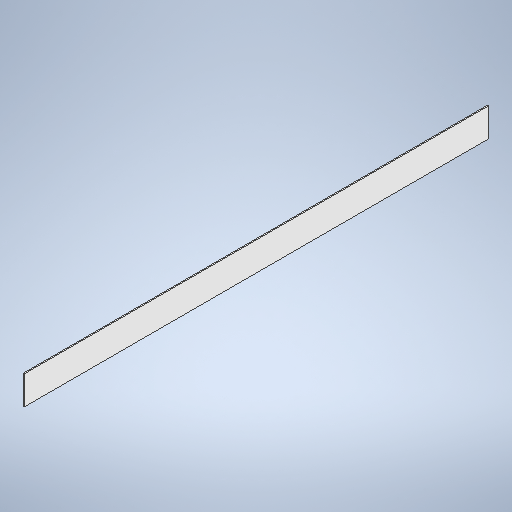
# Autodesk Inventor part: Fiber_Cement_Board_For_Side_Wall
Saved by Autodesk Inventor 2025 (Build 290162010, 162A)
## iProperties
Created: 2024-09-16
Part Number: Fiber_Cement_Board_For_Side_Wall
Material: Generic
Document SubType Name: Modeling
Designer: Tom
Density: 1 g/cm^3
Appearance: White
Author: Tom
Autodesk Inventor part; units mm, degrees
ref_plane "YZ Plane" through (0, 0, 0) normal (1, 0, 0) x (0, 1, 0)
ref_plane "XZ Plane" through (0, 0, 0) normal (0, 1, 0) x (-1, 0, 0)
ref_plane "XY Plane" through (0, 0, 0) normal (0, 0, 1) x (1, 0, 0)
sketch "Sketch1" plane through (0, 0, 0) normal (1, 0, 0) x (0, 1, 0)
  line L0 (0, 0) -> (209.55, 0)
  line L1 (209.55, 0) -> (209.55, 3399.0026)
  line L2 (209.55, 3399.0026) -> (0, 3399.0026)
  line L3 (0, 3399.0026) -> (0, 0)
  dimension "d1" = 209.55
  dimension "d4" = 3399.0026
  constraints: 8 end point, 2 parallel, 1 horizontal, 1 perpendicular
  measures "d1" distance of L0.start L0.end
  measures "d4" distance of L2.end L0.start
extrude "Extrusion1" add sketch "Sketch1" along normal blind 7.9375
body "Solid1"
